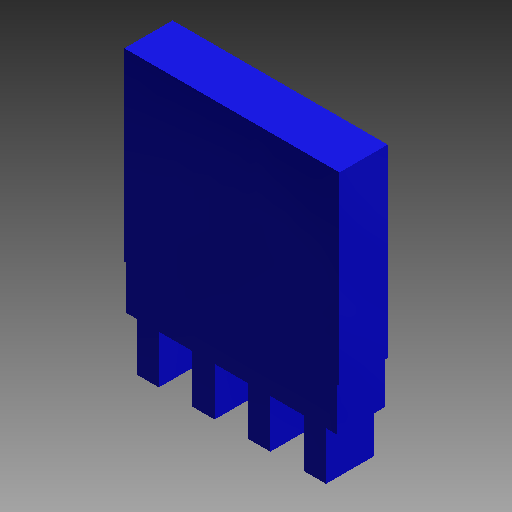
# Autodesk Inventor part: PSMN7R0-60YS,115
Saved by Autodesk Inventor 2018.2 (Build 222227000, 227)
## iProperties
Part Number: PSMN7R0-60YS,115
Material: Generic
Document SubType Name: Modeling
Designer: autocad
Appearance: SOT669, PSMN7R0-60YS,115
Author: autocad
Autodesk Inventor part; units mm, degrees
ref_plane "YZ Plane" through (0, 0, 0) normal (1, 0, 0) x (0, 1, 0)
ref_plane "XZ Plane" through (0, 0, 0) normal (0, 1, 0) x (-1, 0, 0)
ref_plane "XY Plane" through (0, 0, 0) normal (0, 0, 1) x (1, 0, 0)
sketch "SOT669, PSMN7R0-60YS,115_237" plane through (0, 0, 0) normal (0, 0, 1) x (1, 0, 0)
  line L0 (2.4638, -0.96) -> (2.4125, -0.96)
  line L1 (2.4125, -0.96) -> (2.4125, -1.9495)
  line L2 (2.4125, -1.9495) -> (2.159, -1.9495)
  line L3 (2.159, -1.9495) -> (2.159, -3.048)
  line L4 (2.159, -3.048) -> (1.651, -3.048)
  line L5 (1.651, -3.048) -> (1.651, -1.9495)
  line L6 (1.651, -1.9495) -> (0.889, -1.9495)
  line L7 (0.889, -1.9495) -> (0.889, -3.048)
  line L8 (0.889, -3.048) -> (0.381, -3.048)
  line L9 (0.381, -3.048) -> (0.381, -1.9495)
  line L10 (0.381, -1.9495) -> (-0.381, -1.9495)
  line L11 (-0.381, -1.9495) -> (-0.381, -3.048)
  line L12 (-0.381, -3.048) -> (-0.889, -3.048)
  line L13 (-0.889, -3.048) -> (-0.889, -1.9495)
  line L14 (-0.889, -1.9495) -> (-1.651, -1.9495)
  line L15 (-1.651, -1.9495) -> (-1.651, -3.048)
  line L16 (-1.651, -3.048) -> (-2.159, -3.048)
  line L17 (-2.159, -3.048) -> (-2.159, -1.9495)
  line L18 (-2.159, -1.9495) -> (-2.3995, -1.9495)
  line L19 (-2.3995, -1.9495) -> (-2.3995, -0.96)
  line L20 (-2.3995, -0.96) -> (-2.44, -0.96)
  line L21 (-2.44, -0.96) -> (-2.44, 3.2512)
  line L22 (-2.44, 3.2512) -> (2.4638, 3.2512)
  line L23 (2.4638, 3.2512) -> (2.4638, -0.96)
  constraints: 48 end point
extrude "Extrusion1" add sketch "SOT669, PSMN7R0-60YS,115_237" along normal blind 1.1
body "Solid1"
